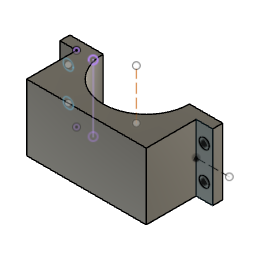
RotaryEncoderStand (Autodesk Fusion 360 design; units mm, degrees)
Autodesk Fusion 360 part; units mm, degrees
sketch "Sketch1" plane through (0, 0, 0) normal (0, 0, 1) x (1, 0, 0)
  line L0 (0, 0) -> (36, 0)
  line L1 (36, 0) -> (36, 18)
  line L2 (36, 18) -> (0, 18)
  line L3 (0, 18) -> (0, 0)
  dimension "d1" = 36
  dimension "d2" = 18
  constraint coincident L0.start L3.end
  constraint horizontal L0
  constraint perpendicular L0 L1
  constraint perpendicular L1 L2
  constraint perpendicular L0 L3
  measures "d1" distance of L0.start L0.end
  measures "d2" distance of L0.end L1.end
extrude "Extrude1" add sketch "Sketch1" along normal blind 20
sketch "Sketch2" plane through (0, 0, 20) normal (0, 0, 1) x (-1, 0, 0)
  line L0 (0, -18) -> (0, 0)
  line L1 (0, 0) -> (-36, 0)
  line L2 (-36, 0) -> (-36, -18)
  line L3 (-36, -18) -> (0, -18)
  circle A0 centre (-18, -18) radius 13
  dimension "d5" = 26
  constraint midpoint L3 A0.centre
  measures "d5" diameter of A0
extrude "Extrude2" cut sketch "Sketch2" against normal blind 20 contours L3 A0 picked at (-19.0768, -11.2377)
ref_plane "WorkPlane1" through (0, 20, 0) normal (0, 1, 0) x (0, 0, 1)
sketch "Sketch3" plane through (36, 0, 0) normal (1, 0, 0) x (0, 1, 0)
  line L0 (0, 0) -> (18, 0)
  line L1 (18, 0) -> (18, 20)
  line L2 (18, 20) -> (0, 20)
  line L3 (0, 20) -> (0, 0)
  line L4 (18, 20) -> (15, 20)
  line L5 (15, 20) -> (15, 0)
  line L6 (15, 0) -> (18, 0)
  line L7 (18, 0) -> (18, 20)
  constraint horizontal L4
  constraint vertical L5
  constraint horizontal L6
  constraint vertical L7
  constraint coincident L0 L5.end
  constraint coincident L1.end L2.start
extrude "Extrude3" add sketch "Sketch3" along normal blind 5 contours L0 L1 L2 L4 L5 L6 L7
sketch "Sketch4" plane through (0, 0, 0) normal (-1, 0, 0) x (0, -1, 0)
  line L0 (-18, 0) -> (0, 0)
  line L1 (0, 0) -> (0, 20)
  line L2 (0, 20) -> (-18, 20)
  line L3 (-18, 20) -> (-18, 0)
  line L4 (-18, 20) -> (-15, 20)
  line L5 (-15, 20) -> (-15, 0)
  line L6 (-15, 0) -> (-18, 0)
  line L7 (-18, 0) -> (-18, 20)
  point P0 (-15, 0)
  constraint horizontal L4
  constraint vertical L5
  constraint horizontal L6
  constraint vertical L7
  constraint coincident P0 L5.end
  constraint coincident L2.end L3.start
extrude "Extrude4" add sketch "Sketch4" along normal blind 5 contours L0 L2 L3 L4 L5 L6 L7
sketch "Sketch5" plane through (0, 15, 0) normal (0, -1, 0) x (1, 0, 0)
  line L0 (36, 20) -> (36, 0)
  line L1 (36, 0) -> (41, 0)
  line L2 (41, 0) -> (41, 20)
  line L3 (41, 20) -> (36, 20)
  line L4 (36, 10) -> (46, 10) construction
  circle A0 centre (38.5, 15) radius 1.5
  line L5 (5, 20) -> (5, 0)
  line L6 (18, 10) -> (18, 25) construction
  circle A1 centre (38.5, 5) radius 1.5
  circle A2 centre (-2.5, 15) radius 1.5
  circle A3 centre (-2.5, 5) radius 1.5
  point P0 (0, 20)
  dimension "d13" = 3
  dimension "d14" = 5
  dimension "d15" = 2.5
  constraint midpoint L0 L4.start
  constraint perpendicular L0 L4
  constraint parallel L5 L6
  constraint symmetric L4 A0 A1
  constraint symmetric A0 L6 A2
  constraint symmetric L6 A1 A3
  measures "d13" diameter of A0
  measures "d14" distance of L3 A0.centre
  measures "d15" distance of L2 A0.centre
